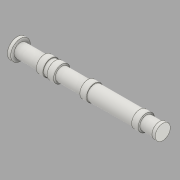
# Autodesk Inventor part: Shaft
Saved by Autodesk Inventor 2020 (Build 240168000, 168)
## iProperties
CustomPartVersion: 1
Created: 2020-08-26
Part Number: Shaft
Material: Steel
Document SubType Name: Modeling
Designer: alons
Density: 1 g/cm^3
Appearance: Steel
Length: 11.100 mm
Author: alons
Autodesk Inventor part; units mm, degrees
ref_plane "Start Plane" through (0, 0, 0) normal (1, 0, 0) x (0, 1, 0)
ref_plane "XZ Plane" through (0, 0, 0) normal (0, 1, 0) x (-1, 0, 0)
sketch "Main Sketch" plane through (0, 0, 0) normal (0, 0, 1) x (1, 0, 0)
  line L0 (0, 0) -> (11.1, 0)
  line L1 (0, 0) -> (0, 0.75)
  line L2 (0, 0.75) -> (0.25, 0.75)
  line L3 (0.25, 0.5) -> (2.082, 0.5)
  line L4 (2.082, 0.575) -> (3.4, 0.575)
  line L5 (3.4, 0.5) -> (5.4, 0.5)
  line L6 (5.4, 0.575) -> (9.85, 0.575)
  line L7 (9.85, 0.5) -> (10.85, 0.5)
  line L8 (11.1, 0.575) -> (11.1, 0)
  line L9 (10.85, 0.575) -> (11.1, 0.575)
  line L10 (0.25, 0.75) -> (0.25, 0.5)
  line L11 (2.082, 0.5) -> (2.082, 0.575)
  line L12 (3.4, 0.575) -> (3.4, 0.5)
  line L13 (5.4, 0.5) -> (5.4, 0.575)
  line L14 (9.85, 0.575) -> (9.85, 0.5)
  line L15 (10.85, 0.5) -> (10.85, 0.575)
  dimension "d3" = 1.5
  dimension "d4" = 1
  dimension "d5" = 1.15
  dimension "d6" = 1
  dimension "d7" = 1.15
  dimension "d8" = 1
  dimension "d9" = 1.15
  constraints: 32 end point, 8 vertical, 2 horizontal
  measures "d3" diameter of L2 L0
  measures "d4" diameter of L3 L0
  measures "d5" diameter of L4 L0
  measures "d6" diameter of L5 L0
  measures "d7" diameter of L6 L0
  measures "d8" diameter of L7 L0
  measures "d9" diameter of L9 L0
revolve "Revolution1" add sketch "Main Sketch" angle 360 about axis through (0, 0, 0) along (1, 0, 0)
ref_plane "Work Plane1" through (2.082, 0, 0) normal (-1, 0, 0) x (0, 0, 1)
sketch "Sketch3" plane through (2.082, 0, 0) normal (-1, 0, 0) x (0, 0, 1)
  circle A0 centre (0, 0) radius 0.575 projected
  circle A1 centre (0, 0) radius 0.75 projected
  circle A2 centre (0, 0) radius 0.625
  dimension "d13" = 1.25
  constraints: 1 centre point, 1 coincident
  measures "d13" diameter of A2
extrude "Extrusion1" add sketch "Sketch3" against normal blind 0.5 contours A2
ref_plane "Work Plane2" through (3.4, 0, 0) normal (-1, 0, 0) x (0, 0, 1)
sketch "Sketch4" plane through (3.4, 0, 0) normal (-1, 0, 0) x (0, 0, 1)
  circle A0 centre (0, 0) radius 0.5 projected
  circle A1 centre (0, 0) radius 0.575 projected
  circle A2 centre (0, 0) radius 0.625
  dimension "d17" = 1.25
  constraints: 1 centre point, 1 coincident
  measures "d17" diameter of A2
extrude "Extrusion2" add sketch "Sketch4" along normal blind 0.5 contours A2
sketch "Sketch5" plane through (5.4, 0, 0) normal (-1, 0, 0) x (0, 0, 1)
  circle A0 centre (0, 0) radius 0.575 projected
  circle A1 centre (0, 0) radius 0.625
  dimension "d20" = 1.25
  constraints: 1 centre point, 1 coincident
  measures "d20" diameter of A1
extrude "Extrusion3" add sketch "Sketch5" against normal blind 0.5
sketch "Sketch6" plane through (9.85, 0, 0) normal (1, 0, 0) x (0, 0, -1)
  circle A0 centre (0, 0) radius 0.625
  circle A1 centre (0, 0) radius 0.575 projected
  dimension "d23" = 1.25
  constraints: 1 centre point, 1 coincident
  measures "d23" diameter of A0
extrude "Extrusion4" add sketch "Sketch6" against normal blind 0.5
equation "\"Length\" = 11.1"
body "Solid1"
